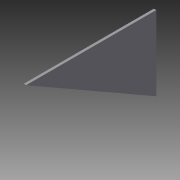
# Autodesk Inventor part: side panel top
Saved by Autodesk Inventor 2015 SP1 (Build 190203100, 203)
## iProperties
Created: 2015-01-28
Part Number: side panel top
Material: Generic
Document SubType Name: Modeling
Designer: Admin
Density: 1 g/cm^3
Appearance: Default
Author: Admin
Autodesk Inventor part; units mm, degrees
ref_plane "YZ Plane" through (0, 0, 0) normal (1, 0, 0) x (0, 1, 0)
ref_plane "XZ Plane" through (0, 0, 0) normal (0, 1, 0) x (-1, 0, 0)
ref_plane "XY Plane" through (0, 0, 0) normal (0, 0, 1) x (1, 0, 0)
sketch "Sketch1" plane through (0, 0, 0) normal (1, 0, 0) x (0, 1, 0)
  line L0 (0, 0) -> (-98.425, 0) construction
  line L1 (-98.425, 0) -> (-98.425, 171.45) construction
  line L2 (-98.425, 171.45) -> (0, 171.45) construction
  line L3 (0, 171.45) -> (0, 0) construction
  line L4 (0, 171.45) -> (0, 0)
  line L5 (0, 0) -> (-98.425, 0)
  line L6 (-98.425, 0) -> (0, 171.45)
  dimension "d0" = 98.425
  dimension "d1" = 171.45
  constraints: 14 end point, 3 equal length, 2 perpendicular, 1 horizontal
  measures "d0" distance of L1.end L2.end
  measures "d1" distance of L0.end L1.end
extrude "Extrusion1" add sketch "Sketch1" along normal blind 3.175
body "Solid1"
